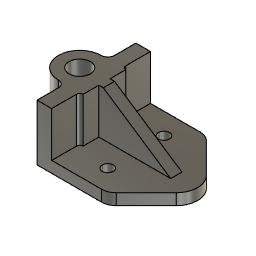
A3 (Autodesk Fusion 360 design; units mm, degrees)
Autodesk Fusion 360 part; units mm, degrees
sketch "Sketch1" plane through (0, 0, 0) normal (0, 0, 1) x (1, 0, 0)
  line L0 (0, 44) -> (67, 44)
  line L1 (67, -44) -> (0, -44)
  line L2 (0, 0) -> (67, 0) construction
  line L3 (0, 44) -> (0, -44)
  line L4 (80.435, -13.435) -> (49.8701, -44)
  line L5 (80.435, 13.435) -> (49.8701, 44)
  arc A0 (80.435, -13.435) -> (80.435, 13.435) centre (67, 0) ccw
  dimension "d2" = 67
  dimension "d3" = 88
  dimension "d4" = 67
  dimension "d6" = 38
  dimension "d9" = 45
  dimension "d10" = 45
  constraint symmetric L0 L1 L2
  constraint coincident L2.end A0.centre
  constraint coincident L1 L4.end
  constraint coincident L0 L5.end
  constraint tangent L4 A0
  constraint tangent L5 A0
  constraint coincident origin L2
  constraint coincident L2.start L3
  measures "d2" distance of L0.start L0.end
  measures "d3" distance of L0.end L1.start
  measures "d4" distance of L1.start L1.end
  measures "d6" diameter of A0
  measures "d9" angle of L2 L4
  measures "d10" angle of L2 L5
extrude "Extrude2" add sketch "Sketch1" along normal blind 10
sketch "Sketch5" plane through (0, 0, 10) normal (0, 0, 1) x (-1, 0, 0)
  line L0 (-49.8701, 44) -> (-80.435, 13.435)
  arc A0 (-80.435, 13.435) -> (-80.435, -13.435) centre (-67, 0) ccw
  line L1 (-80.435, -13.435) -> (-49.8701, -44)
  line L2 (-49.8701, -44) -> (0, -44)
  line L3 (0, -44) -> (0, 44)
  line L4 (0, 44) -> (-49.8701, 44)
  line L5 (0, -44) -> (13, -44)
  line L6 (13, -44) -> (13, -19)
  line L7 (13, -19) -> (19, -19)
  line L8 (19, 0) -> (0, 0) construction
  line L9 (0, 44) -> (13, 44)
  line L10 (13, 44) -> (13, 19)
  line L11 (13, 19) -> (19, 19)
  arc A1 (19, -19) -> (19, 19) centre (19, 0) ccw
  line L12 (0, -19) -> (-3, -19)
  line L13 (-3, -19) -> (-3, -5)
  line L14 (-3, -5) -> (-7, -5)
  line L15 (-7, -5) -> (-7, 0)
  line L16 (0, 19) -> (-3, 19)
  line L17 (-3, 19) -> (-3, 5)
  line L18 (-3, 5) -> (-7, 5)
  line L19 (-7, 5) -> (-7, 0)
  line L20 (0, -44) -> (0, -19)
  line L21 (0, 19) -> (0, 44)
  dimension "d15" = 13
  dimension "d16" = 38
  dimension "d17" = 6
  dimension "d18" = 3
  dimension "d19" = 14
  dimension "d20" = 4
  constraint coincident L2.end L3.start
  constraint perpendicular L3 L5
  constraint perpendicular L5 L6
  constraint perpendicular L3 L7
  constraint tangent L7 A1
  constraint coincident L8.start A1.centre
  constraint perpendicular L3 L8
  constraint symmetric L2.end L8 L3.end
  constraint symmetric L5.end L8 L9.end
  constraint symmetric L6.end L8 L10.end
  constraint symmetric L7.end L8 L11.end
  constraint coincident L3.end L4.start
  constraint coincident L3 L12.start
  constraint perpendicular L3 L12
  constraint perpendicular L8 L13
  constraint perpendicular L13 L14
  constraint perpendicular L8 L15
  constraint symmetric L8 L12.start L16.start
  constraint symmetric L8 L12.end L16.end
  constraint symmetric L8 L13.end L17.end
  constraint symmetric L8 L14.end L18.end
  constraint symmetric L8 L15.end L19.end
  constraint collinear L20 L21
  measures "d15" distance of L2.end L5.end
  measures "d16" diameter of A1
  measures "d17" distance of L6.end L7.end
  measures "d18" distance of L16.start L16.end
  measures "d19" distance of L16.end L17.end
  measures "d20" distance of L17.end L18.end
extrude "Extrude4" add sketch "Sketch5" along normal blind 40 contours L3 L12 L13 L14 L15 L16 L17 L18 L19
extrude "Extrude3" add sketch "Sketch5" along normal blind 40 and the other way blind 10 contours L3 L5 L6 L7 L9 L10 L11 A1 L20 L21
ref_plane "WorkPlane1" through (18.435, 0, 25) normal (0, 1, 0) x (-1, 0, 0)
sketch "Sketch7" plane through (7, 0, 0) normal (1, 0, 0) x (0, 1, 0)
  line L0 (-5, 10) -> (5, 10)
  line L1 (5, 10) -> (5, 50)
  line L2 (5, 50) -> (-5, 50)
  line L3 (-5, 50) -> (-5, 10)
  line L4 (0, 50) -> (0, 10) construction
  constraint midpoint L0 L4.end
  constraint perpendicular L0 L4
sketch "Sketch8" plane through (0, 0, 10) normal (0, 0, 1) x (-1, 0, 0)
  line L0 (-47, 36) -> (-47, -54) construction
  line L1 (-47, -9) -> (-3.8729, -9) construction
  line L2 (-47, -9) -> (-47, -34) construction
  line L3 (-47, -9) -> (-11, -9) construction
  line L4 (-67, 44) -> (-67, -44) construction
  line L5 (-67, -9) -> (-67, -34) construction
  line L6 (-67, -9) -> (-31, -9) construction
  line L7 (-67, 0) -> (-7.0889, 0) construction
  line L8 (-31, 0) -> (-31, -25) construction
  line L9 (-31, 0) -> (-31, 25) construction
  point P0 (-67, 44)
  point P1 (-67, -44)
  dimension "d37" = 25
  dimension "d39" = 36
  dimension "d45" = 25
  dimension "d49" = 25
  constraint vertical L0
  constraint midpoint L0 L1.start
  constraint perpendicular L0 L1
  constraint perpendicular L1 L2
  constraint perpendicular L0 L3
  constraint perpendicular L3 L4
  constraint coincident L4 L5.start
  constraint coincident L4 L5.end
  constraint perpendicular L0 L6
  constraint coincident P0 L4.start
  constraint coincident P1 L4.end
  constraint midpoint L4 L7.start
  constraint perpendicular L0 L7
  constraint coincident L7 L8.start
  constraint perpendicular L6 L8
  constraint perpendicular L7 L9
  measures "d37" distance of L1.start L2.end
  measures "d39" distance of L5.start L6.end
  measures "d45" distance of L8.start L8.end
  measures "d49" distance of L8.start L9.end
sketch "Sketch6" plane through (18.435, 0, 25) normal (0, 1, 0) x (1, 0, 0)
  line L0 (-11.435, 15) -> (-11.435, -25)
  line L1 (-11.435, -25) -> (48.565, 15)
  line L2 (48.565, 15) -> (-11.435, 15)
  point P0 (-11.435, 15)
  point P1 (-11.435, -25)
  point P2 (48.565, 15)
  constraint coincident L0 P0
  constraint coincident L0.end L1.start
  constraint perpendicular L0 L2
  constraint coincident P2 L1.end
extrude "Extrude6" add sketch "Sketch6" along normal mid plane 10
hole "Hole2" at (-19, 0, 50) direction (0, 0, -1) diameter 19 depth 50 tip angle 118
hole "Hole3" at (31, 25, 10) direction (0, 0, -1) diameter 10 depth 50 tip angle 118
hole "Hole4" at (31, -25, 10) direction (0, 0, -1) diameter 10 depth 50 tip angle 118
fillet "Fillet7" radius 13 2 edges at (49.8701, -44, 5) (49.8701, 44, 5)
fillet "Fillet8" radius 3 2 edges at (0, 19, 30) (0, -19, 30)
fillet "Fillet9" radius 6 2 edges at (-13, -19, 25) (-13, 19, 25)
extrude "Extrude5" [suppressed]
fillet "Fillet3" [suppressed]
fillet "Fillet4" [suppressed]
fillet "Fillet5" [suppressed]
fillet "Fillet6" [suppressed]
sketch "Sketch9" plane through (0, 0, 50) normal (0, 0, 1) x (-1, 0, 0)
  line L0 (-3, 19) -> (-3, 5)
  line L1 (-3, 5) -> (-7, 5)
  line L2 (-7, -5) -> (-3, -5)
  line L3 (-3, -5) -> (-3, -19)
  arc A0 (0, -22) -> (-3, -19) centre (-3, -22) ccw
  line L4 (0, -22) -> (0, -44)
  line L5 (0, -44) -> (13, -44)
  line L6 (13, -44) -> (13, -25)
  arc A1 (19, -19) -> (13, -25) centre (19, -25) ccw
  arc A2 (19, -19) -> (19, 19) centre (19, 0) ccw
  arc A3 (13, 25) -> (19, 19) centre (19, 25) ccw
  line L7 (13, 25) -> (13, 44)
  line L8 (13, 44) -> (0, 44)
  line L9 (0, 44) -> (0, 22)
  arc A4 (-3, 19) -> (0, 22) centre (-3, 22) ccw
  circle A5 centre (19, 0) radius 9.5 construction
  line L10 (-7, 5) -> (-7, 0)
  line L11 (-7, 0) -> (-7, -5)
  dimension "d33" = 19
  constraint concentric A2 A5
  measures "d33" diameter of A5
hole "Hole1" [suppressed]
